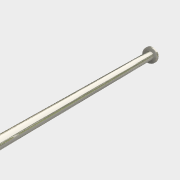
# Autodesk Inventor part: PWTR-0137
Saved by Autodesk Inventor 2021.1 (Build 251245000, 245)
## iProperties
Created: 2020-09-01
Part Number: PWTR-0137
Material: Stainless Steel
Document SubType Name: Modeling
Designer: alid
Density: 8 g/cm^3
Appearance: Titanium - Polished
Description: Arm Pivot Pin
Author: alid
Revision Number: A
Autodesk Inventor part; units mm, degrees
note: some values were not read from the file. Chosen so that the rebuilt part matches the saved one: edges of "Chamfer1".
ref_plane "YZ Plane" through (0, 0, 0) normal (1, 0, 0) x (0, 1, 0)
ref_plane "XZ Plane" through (0, 0, 0) normal (0, 1, 0) x (-1, 0, 0)
ref_plane "XY Plane" through (0, 0, 0) normal (0, 0, 1) x (1, 0, 0)
sketch "Sketch1" plane through (0, 0, 0) normal (0, 0, 1) x (1, 0, 0)
  line L0 (-148.0565, 0) -> (148.0565, 0)
  line L1 (-148.0565, 0) -> (-148.0565, 8)
  line L2 (-148.0565, 8) -> (143.0565, 8)
  line L3 (143.0565, 8) -> (143.0565, 15)
  line L4 (143.0565, 15) -> (148.0565, 15)
  line L5 (148.0565, 15) -> (148.0565, 0)
  circle A0 centre (-143.0565, 0) radius 1.75
  point P0 (0, 0)
  point P1 (0, 0)
  point P2 (143.0565, 8.25)
  dimension "d0" = 296.113
  dimension "d1" = 16
  dimension "d2" = 5
  dimension "d3" = 30
  dimension "d8" = 3.5
  dimension "d9" = 5
  dimension "d12" = 0.25
  constraints: 12 end point, 4 perpendicular, 2 point on line, 1 centre point, 1 coincident, 1 horizontal, 1 midpoint, 1 vertical
  measures "d0" distance of L0.start L0.end
  measures "d1" diameter of L2 L0
  measures "d2" distance of L3.end L4.end
  measures "d3" diameter of L4 L0
  measures "d8" diameter of A0
  measures "d9" distance from line of L1 A0.centre
  measures "d12" distance from line of L2 point (143.056, 8.25)
revolve "Revolution1" add sketch "Sketch1" angle 360 about axis through (-148.0565, 0, 0) along (1, 0, 0) picked at (-142.9862, 0.5791) contours A0 L0 L1 L2 L3 L4 L5 | L0 A0
fillet "Fillet1" radius 1 1 edges at (-148.0565, -8, 0)
chamfer "Chamfer1" distance 1 angle 45 3 edges at (148.0565, -15, 0) (-147.0565, -8, 0) (-148.0565, -7, 0)
extrude "Extrusion2" cut sketch "Sketch1" against normal through all both and the other way through all contours A0 L0 | L0 A0
body "Solid1"
